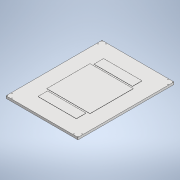
# Autodesk Inventor part: base_plate
Saved by Autodesk Inventor 2021 (Build 250183000, 183)
## iProperties
Created: 2023-01-13
Part Number: base_plate
Material: Типовые
Document SubType Name: Modeling
Designer: ignat
Density: 1 g/cm^3
Appearance: По умолчанию
Author: ignat
Autodesk Inventor part; units mm, degrees
ref_plane "YZ Plane" through (0, 0, 0) normal (1, 0, 0) x (0, 1, 0)
ref_plane "XZ Plane" through (0, 0, 0) normal (0, 1, 0) x (-1, 0, 0)
ref_plane "XY Plane" through (0, 0, 0) normal (0, 0, 1) x (1, 0, 0)
sketch "Эскиз1" plane through (0, 0, 0) normal (0, 1, 0) x (-1, 0, 0)
  line L0 (-225, 300) -> (225, 300)
  line L1 (225, 300) -> (225, -300)
  line L2 (225, -300) -> (-225, -300)
  line L3 (-225, -300) -> (-225, 300)
  line L4 (-225, 300) -> (225, -300) construction
  line L5 (225, 300) -> (-225, -300) construction
  line L6 (-135, 135) -> (135, 135)
  line L7 (135, 135) -> (135, -135)
  line L8 (135, -135) -> (-135, -135)
  line L9 (-135, -135) -> (-135, 135)
  line L10 (-135, 135) -> (135, -135) construction
  line L11 (135, 135) -> (-135, -135) construction
  line L12 (120, 145) -> (-120, 145)
  line L13 (-120, 145) -> (-120, 205)
  line L14 (-120, 205) -> (120, 205)
  line L15 (120, 205) -> (120, 145)
  line L16 (120, -145) -> (-120, -145)
  line L17 (-120, -145) -> (-120, -205)
  line L18 (-120, -205) -> (120, -205)
  line L19 (120, -205) -> (120, -145)
  point P0 (0, 0)
  dimension "d0" = 450
  dimension "d1" = 600
  dimension "d2" = 270
  dimension "d3" = 270
  dimension "d7" = 240
  dimension "d8" = 60
  dimension "d9" = 60
  dimension "d10" = 15
  dimension "d11" = 10
  dimension "d12" = 10
  dimension "d13" = 15
  constraints: 40 end point, 8 parallel, 4 horizontal, 4 midpoint, 4 perpendicular, 2 point on line
  measures "d0" distance of L1.end L2.end
  measures "d1" distance of L0.end L1.end
  measures "d2" distance of L7.end L8.end
  measures "d3" distance of L6.end L7.end
  measures "d7" distance of L13.end L14.end
  measures "d8" distance of L12.end L13.end
  measures "d9" distance of L17.end L16.end
  measures "d10" distance between parallel lines of L7 L15
  measures "d11" distance between parallel lines of L6 L12
  measures "d12" distance between parallel lines of L8 L16
  measures "d13" distance between parallel lines of L7 L19
extrude "Выдавливание1" add sketch "Эскиз1" along normal blind 14
extrude "Выдавливание2" add sketch "Эскиз1" along normal blind 15.5 contours L6 L7 L8 L9 | L12 L13 L14 L15 | L19 L18 L17 L16
sketch "Эскиз2" plane through (0, 14, 0) normal (0, 1, 0) x (1, 0, 0)
  circle A0 centre (-193.75, 293.75) radius 1.75
  circle A1 centre (-218.75, 268.75) radius 1.75
  circle A2 centre (-221, 296) radius 1.75
  circle A3 centre (221, 296) radius 1.75
  circle A4 centre (218.75, 268.75) radius 1.75
  circle A5 centre (193.75, 293.75) radius 1.75
  circle A6 centre (218.75, -268.75) radius 1.75
  circle A7 centre (221, -296) radius 1.75
  circle A8 centre (193.75, -293.75) radius 1.75
  circle A9 centre (-218.75, -268.75) radius 1.75
  circle A10 centre (-221, -296) radius 1.75
  circle A11 centre (-193.75, -293.75) radius 1.75
  line L0 (225, 300) -> (-225, 300) projected
  line L1 (-225, 300) -> (-225, -300) projected
  line L2 (225, -300) -> (225, 300) projected
  line L3 (-225, -300) -> (225, -300) projected
  point P0 (0, 0)
  dimension "d20" = 27.25
  dimension "d21" = 27.25
  dimension "d22" = 2.25
  dimension "d23" = 2.25
  dimension "d24" = 4
  dimension "d25" = 4
  dimension "d26" = 27.25
  dimension "d27" = 27.25
  dimension "d28" = 2.25
  dimension "d29" = 2.25
  dimension "d30" = 4
  dimension "d31" = 4
  dimension "d32" = 27.25
  dimension "d33" = 27.25
  dimension "d34" = 2.25
  dimension "d35" = 2.25
  dimension "d36" = 4
  dimension "d37" = 4
  dimension "d38" = 27.25
  dimension "d39" = 27.25
  dimension "d40" = 2.25
  dimension "d41" = 2.25
  dimension "d42" = 4
  dimension "d43" = 4
  constraints: 12 centre point
  measures "d20" horizontal distance of A0.centre A2.centre
  measures "d21" vertical distance of A2.centre A1.centre
  measures "d22" horizontal distance of A1.centre A2.centre
  measures "d23" vertical distance of A0.centre A2.centre
  measures "d24" distance from line of L0 A2.centre
  measures "d25" distance from line of L1 A2.centre
  measures "d26" horizontal distance of A3.centre A5.centre
  measures "d27" vertical distance of A4.centre A3.centre
  measures "d28" horizontal distance of A3.centre A4.centre
  measures "d29" vertical distance of A5.centre A3.centre
  measures "d30" distance from line of L0 A3.centre
  measures "d31" distance from line of A3.centre L2
  measures "d32" horizontal distance of A8.centre A7.centre
  measures "d33" vertical distance of A6.centre A7.centre
  measures "d34" vertical distance of A8.centre A7.centre
  measures "d35" horizontal distance of A6.centre A7.centre
  measures "d36" distance from line of L3 A7.centre
  measures "d37" distance from line of A7.centre L2
  measures "d38" horizontal distance of A11.centre A10.centre
  measures "d39" vertical distance of A9.centre A10.centre
  measures "d40" horizontal distance of A9.centre A10.centre
  measures "d41" vertical distance of A11.centre A10.centre
  measures "d42" distance from line of L3 A10.centre
  measures "d43" distance from line of L1 A10.centre
extrude "Выдавливание3" cut sketch "Эскиз2" against normal through all contours A0 | A1 | A2 | A3 | A4 | A5 | A6 | A7 | A8 | A9 | A10 | A11
